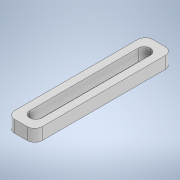
# Autodesk Inventor part: extention_plate
Saved by Autodesk Inventor 2020 (Build 240168000, 168)
## iProperties
Created: 2019-09-23
Part Number: extention_plate
Material: Generic
Document SubType Name: Modeling
Designer: dlr6513
Density: 1 g/cm^3
Appearance: Default
Author: dlr6513
Autodesk Inventor part; units mm, degrees
ref_plane "YZ Plane" through (0, 0, 0) normal (1, 0, 0) x (0, 1, 0)
ref_plane "XZ Plane" through (0, 0, 0) normal (0, 1, 0) x (-1, 0, 0)
ref_plane "XY Plane" through (0, 0, 0) normal (0, 0, 1) x (1, 0, 0)
sketch "Sketch1" plane through (0, 0, 0) normal (0, 1, 0) x (-1, 0, 0)
  line L0 (16.3851, 33.9368) -> (4.9404, 33.9368)
  line L1 (4.9404, 33.9368) -> (4.9404, -23.2869)
  line L2 (4.9404, -23.2869) -> (16.3851, -23.2869)
  line L3 (16.3851, -23.2869) -> (16.3851, 33.9368)
  line L4 (13.2127, 30.325) -> (8.1127, 30.325)
  line L5 (8.1127, 30.325) -> (8.1127, -19.675)
  line L6 (8.1127, -19.675) -> (13.2127, -19.675)
  line L7 (13.2127, -19.675) -> (13.2127, 30.325)
  point P0 (0, 0)
  dimension "d2" = 5.1
  dimension "d3" = 11.4447
  dimension "d4" = 57.2237
  dimension "d5" = 3.1724
  dimension "d6" = 50
  dimension "d7" = 3.6118
  constraints: 16 end point, 4 parallel, 2 horizontal, 2 perpendicular
  measures "d2" distance between parallel lines of L5 L7
  measures "d3" distance of L1.end L2.end
  measures "d4" distance of L2.end L0.start
  measures "d5" distance between parallel lines of L3 L7
  measures "d6" distance of L6.end L4.start
  measures "d7" distance between parallel lines of L0 L4
extrude "Extrusion1" add sketch "Sketch1" along normal blind 5
fillet "Fillet1" radius 2.54 4 edges at (-8.1127, 2.5, -19.675) (-13.2127, 2.5, -19.675) (-13.2127, 2.5, 30.325) (-8.1127, 2.5, 30.325)
fillet "Fillet2" radius 3.175 4 edges at (-16.3851, 2.5, 33.9368) (-4.9404, 2.5, 33.9368) (-16.3851, 2.5, -23.2869) (-4.9404, 2.5, -23.2869)
equation "\"d5\" = -0.5 * d2 + 0.5 * d3"
equation "\"d7\" = -0.5 * d6 + 0.5 * d4"
body "Solid1"
